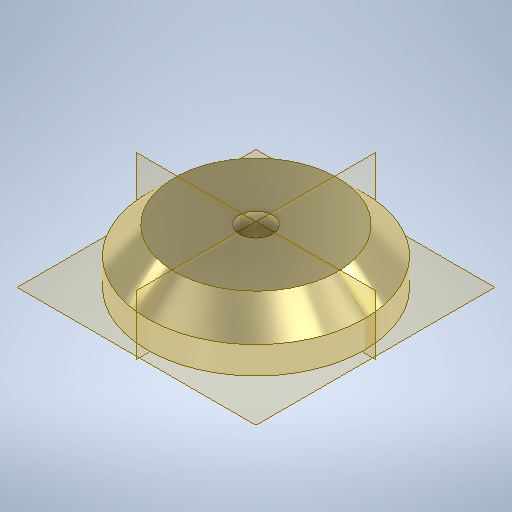
# Autodesk Inventor part: Sessao9__08_04_2025_0001_001
Saved by Autodesk Inventor 2025.2 (Build 292293000, 293)
## iProperties
Created: 2025-04-08
Part Number: Sessao9__08_04_2025_0001_001
Material: Ouro
Document SubType Name: Modeling
Designer: Gustavo Sousa
Density: 19.3 g/cm^3
Appearance: Ouro - Metal
Author: Gustavo Sousa
Autodesk Inventor part; units mm, degrees
sketch "Esboço1" plane through (0, 0, 0) normal (0, 0, 1) x (1, 0, 0)
  line L0 (-40, 0) -> (-40, 10)
  line L1 (-40, 10) -> (-30, 20)
  line L2 (-30, 20) -> (0, 20)
  line L3 (-40, 0) -> (0, 0)
  line L4 (0, 20) -> (0, 0)
  line L5 (0, -4) -> (0, 24) projected
  dimension "d0" = 40
  dimension "d1" = 10
  dimension "d6" = 135
  dimension "d7" = 30
  constraints: 10 end point, 2 vertical, 1 horizontal, 1 horizontal alignment, 1 vertical alignment
  measures "d0" distance from line of L3.end L0
  measures "d1" distance of L0.start L0.end
  measures "d6" angle of L0 L1
  measures "d7" distance of L1.end L2.end
revolve "Revolução1" add sketch "Esboço1" angle 360 mid plane about axis through (0, -10, 0) along (0, 1, 0)
sketch "Esboço2" plane through (0, 20, 0) normal (0, 1, 0) x (1, 0, 0)
  circle A0 centre (0, 0) radius 6.1
  dimension "d9" = 12.2
  constraints: 1 centre point, 1 coincident
  measures "d9" diameter of A0
extrude "Extrusão1" cut sketch "Esboço2" against normal blind 10
